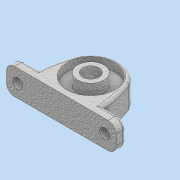
# Autodesk Inventor part: Łożysko w obudowie aluminiowej 10mm KP000
Saved by Autodesk Inventor 2018 (Build 220112000, 112)
## iProperties
Created: 2019-01-23
Part Number: Łożysko w obudowie aluminiowej 10mm KP000
Material: Ogólny
Document SubType Name: Modeling
Designer: Dawid
Density: 1 g/cm^3
Appearance: Aluminium odlewane
Author: Dawid
Autodesk Inventor part; units mm, degrees
ref_plane "YZ Plane" through (0, 0, 0) normal (1, 0, 0) x (0, 1, 0)
ref_plane "XZ Plane" through (0, 0, 0) normal (0, 1, 0) x (-1, 0, 0)
sketch "Szkic1" plane through (0, 0, 0) normal (0, 0, 1) x (1, 0, 0)
  line L0 (0, 0) -> (33.5, 0)
  line L1 (0, 0) -> (-33.5, 0)
  circle A0 centre (0, 18) radius 5
  line L2 (-33.5, 0) -> (-33.5, 6)
  line L3 (33.5, 6) -> (33.5, 0)
  line L4 (-19.5, 6) -> (-26.5, 6)
  line L5 (19.5, 6) -> (26.5, 6)
  line L6 (-26.5, 6) -> (-19.5, 6)
  line L7 (26.5, 6) -> (19.5, 6)
  line L8 (0, 18) -> (-14.722432, 26.5) construction
  line L9 (0, 18) -> (0, 35) construction
  line L10 (0, 18) -> (14.722432, 26.5) construction
  line L11 (0, 18) -> (0, 35) construction
  arc A1 (19.5, 6) -> (14.722432, 26.5) centre (-44.369926, 1.921691) ccw
  line L12 (-33.5, 6) -> (-19.5, 6)
  line L13 (19.5, 6) -> (33.5, 6)
  arc A2 (-14.722432, 26.5) -> (-19.5, 6) centre (44.369926, 1.921691) ccw
  line L14 (-19.5, 6) -> (19.5, 6)
  line L15 (-14.722432, 26.5) -> (-14.722432, 6)
  line L16 (14.722432, 26.5) -> (14.722432, 6)
  arc A3 (0, 35) -> (-14.722432, 26.5) centre (0, 18) ccw
  arc A4 (14.722432, 26.5) -> (0, 35) centre (0, 18) ccw
  dimension "d0" = 33.5
  dimension "d1" = 33.5
  dimension "d2" = 35
  dimension "d4" = 10
  dimension "d5" = 6
  dimension "d9" = 7
  dimension "d10" = 7
  dimension "d11" = 60
  dimension "d12" = 60
  dimension "d14" = 64
  dimension "d15" = 64
  constraints: 34 end point, 9 point on circle, 5 centre point, 4 coincident, 4 point on line, 2 midpoint, 2 perpendicular, 1 horizontal
  measures "d0" distance of L0.start L0.end
  measures "d1" distance of L0.start L1.end
  measures "d2" distance of L0.start L9.end
  measures "d4" diameter of A0
  measures "d5" distance of L1.end L2.end
  measures "d9" distance of L4.start L4.end
  measures "d10" distance of L5.start L5.end
  measures "d11" angle of L9 L8
  measures "d12" angle of L10 L11
  measures "d14" radius of A1
  measures "d15" radius of A2
sketch "Szkic1 outline for Wyciągnięcie proste1" plane through (0, 0, 0) normal (0, 0, 1) x (1, 0, 0)
  arc A0 (19.5, 6) -> (14.722432, 26.5) centre (-44.369926, 1.921691) ccw
  arc A1 (14.722432, 26.5) -> (-14.722432, 26.5) centre (0, 18) ccw
  arc A2 (-14.722432, 26.5) -> (-19.5, 6) centre (44.369926, 1.921691) ccw
  line L0 (-19.5, 6) -> (-33.5, 6)
  line L1 (-33.5, 6) -> (-33.5, 0)
  line L2 (-33.5, 0) -> (33.5, 0)
  line L3 (33.5, 0) -> (33.5, 6)
  line L4 (33.5, 6) -> (19.5, 6)
  circle A3 centre (0, 18) radius 5
extrude "Wyciągnięcie proste1" add sketch "Szkic1 outline for Wyciągnięcie proste1" along normal blind 16
sketch "Szkic2" plane through (-33.5, 0, 0) normal (0, -1, 0) x (1, 0, 0)
  circle A0 centre (7, 8) radius 3
  circle A1 centre (60, 8) radius 3
  constraints: 2 centre point
sketch "Szkic2 outline for Wyciągnięcie proste2" plane through (-33.5, 0, 0) normal (0, -1, 0) x (1, 0, 0)
  circle A0 centre (7, 8) radius 3
  circle A1 centre (60, 8) radius 3
extrude "Wyciągnięcie proste2" cut sketch "Szkic2 outline for Wyciągnięcie proste2" against normal up to next
ref_plane "Płaszczyzna konstrukcyjna1" through (0, 0, 8) normal (0, 0, 1) x (1, 0, 0)
sketch "Szkic3" plane through (0, 0, 8) normal (0, 0, 1) x (1, 0, 0)
  circle A0 centre (0, 18) radius 5 projected
  circle A1 centre (0, 18) radius 8
  point P0 (0, 0)
  dimension "d28" = 16
  constraints: 1 centre point, 1 coincident
  measures "d28" diameter of A1
sketch "Szkic3 outline for Wyciągnięcie proste3" plane through (0, 0, 8) normal (0, 0, 1) x (1, 0, 0)
  circle A0 centre (0, 18) radius 8
  circle A1 centre (0, 18) radius 5
extrude "Wyciągnięcie proste3" add sketch "Szkic3 outline for Wyciągnięcie proste3" along normal blind 10
sketch "Szkic4" plane through (0, 0, 16) normal (0, 0, 1) x (1, 0, 0)
  arc A0 (-14.722432, 26.5) -> (-19.5, 6) centre (44.369926, 1.921691) ccw
  arc A1 (14.722432, 26.5) -> (-14.722432, 26.5) centre (0, 18) ccw
  arc A2 (19.5, 6) -> (14.722432, 26.5) centre (-44.369926, 1.921691) ccw
  arc A3 (-16.750014, 20.904656) -> (16.750014, 20.904656) centre (0, 18) ccw
  circle A4 centre (0, 18) radius 14.5
  circle A5 centre (0, 18) radius 8
  point P0 (0, 0)
  dimension "d31" = 29
  constraints: 10 point on circle, 5 centre point, 2 coincident
  measures "d31" diameter of A4
sketch "Szkic4 outline for Wyciągnięcie proste4" plane through (0, 0, 16) normal (0, 0, 1) x (1, 0, 0)
  circle A0 centre (0, 18) radius 14.5
  circle A1 centre (0, 18) radius 8
extrude "Wyciągnięcie proste4" cut sketch "Szkic4 outline for Wyciągnięcie proste4" against normal blind 5
sketch "Szkic5" plane through (0, 0, 0) normal (0, 0, -1) x (-1, 0, 0)
  circle A0 centre (0, 18) radius 5
  circle A1 centre (0, 18) radius 8
  arc A2 (14.722432, 26.5) -> (-14.722432, 26.5) centre (0, 18) ccw
  arc A3 (19.5, 6) -> (14.722432, 26.5) centre (-44.369926, 1.921691) ccw
  arc A4 (-14.722432, 26.5) -> (-19.5, 6) centre (44.369926, 1.921691) ccw
  arc A5 (-14.722432, 26.5) -> (-19.5, 6) centre (44.369926, 1.921691) ccw
  arc A6 (19.5, 6) -> (14.722432, 26.5) centre (-44.369926, 1.921691) ccw
  arc A7 (-16.750014, 20.904656) -> (16.750014, 20.904656) centre (0, 18) ccw
  circle A8 centre (0, 18) radius 14.5
  point P0 (0, 0)
  dimension "d34" = 16
  dimension "d35" = 29
  constraints: 14 point on circle, 9 centre point, 3 coincident
  measures "d34" diameter of A1
  measures "d35" diameter of A8
sketch "Szkic5 outline for Wyciągnięcie proste5" plane through (0, 0, 0) normal (0, 0, -1) x (-1, 0, 0)
  circle A0 centre (0, 18) radius 14.5
  circle A1 centre (0, 18) radius 8
extrude "Wyciągnięcie proste5" cut sketch "Szkic5 outline for Wyciągnięcie proste5" against normal blind 5
sketch "Szkic6" plane through (0, 18, 0) normal (0, 0, -1) x (-1, 0, 0)
  circle A0 centre (0, 0) radius 8 projected
  circle A1 centre (0, 0) radius 5 projected
  point P0 (0, -18)
sketch "Szkic6 outline for Wyciągnięcie proste6" plane through (0, 18, 0) normal (0, 0, -1) x (-1, 0, 0)
  circle A0 centre (0, 0) radius 8
  circle A1 centre (0, 0) radius 5
extrude "Wyciągnięcie proste6" cut sketch "Szkic6 outline for Wyciągnięcie proste6" against normal blind 4
fillet "Zaokrąglenie1" radius 5 4 edges at (-33.5, 3, 16) (-33.5, 3, 0) (33.5, 3, 16) (33.5, 3, 0)
fillet "Zaokrąglenie2" radius 2 14 edges at (17.9598, 16.4478, 16) (0, 35, 16) (-17.9598, 16.4478, 16) (32.0355, 6, 14.5355) (33.5, 6, 8) (32.0355, 6, 1.4645) (-24, 6, 0) (24, 6, 16) (-32.0355, 6, 14.5355) (-33.5, 6, 8) (-32.0355, 6, 1.4645) (0, 35, 0) (-17.9598, 16.4478, 0) (17.9598, 16.4478, 0)
